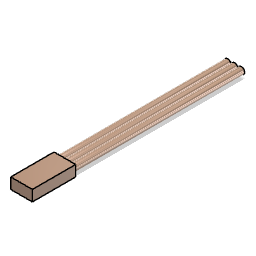
1,2 of P7-501 thermal strap v2 (Autodesk Fusion 360 design; units mm, degrees)
Autodesk Fusion 360 part; units mm, degrees
sketch "Sketch1" plane through (0, 0, 0) normal (0, 1, 0) x (1, 0, 0)
  line L0 (-6.35, 25.4) -> (6.35, 25.4)
  line L1 (6.35, 25.4) -> (6.35, 0)
  line L2 (6.35, 0) -> (-6.35, 0)
  line L3 (-6.35, 0) -> (-6.35, 25.4)
  line L4 (-4, 25.4) -> (-4, 125)
  line L5 (-4, 125) -> (-2, 125)
  line L6 (-2, 125) -> (-2, 25.4)
  dimension "d1" = 25.4
  dimension "d2" = 12.7
  dimension "d5" = 125
  dimension "d6" = 2
  dimension "d12" = 2
  constraint horizontal L0
  constraint vertical L1
  constraint horizontal L2
  constraint vertical L3
  constraint midpoint origin L2
  constraint perpendicular L0 L4
  constraint perpendicular L4 L5
  constraint coincident L0 L6.end
  constraint perpendicular L0 L6
  constraint coincident L0 L4.start
  measures "d1" distance of L0.start L2.end
  measures "d2" distance of L1.end L2.end
  measures "d5" distance of L2 L5
  measures "d6" distance of L4 L6
  measures "d12" distance of origin L6
extrude "Extrude1" add sketch "Sketch1" along normal mid plane 6.35 contours L0 L1 L2 L3
revolve "Revolve1" add sketch "Sketch1" angle 360 about axis through (-4, 0, -25.4) along (0, 0, -1) contours L0 L4 L5 L6
pattern_linear "R-Pattern1" count 3 spacing 4 along (1, 0, 0) of "Revolve1"
